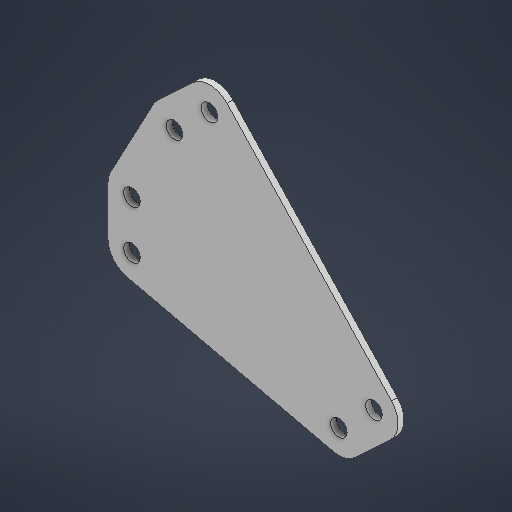
# Autodesk Inventor part: 2-Gearbox
Saved by Autodesk Inventor 2026.1 (Build 301233000, 233)
## iProperties
Created: 2025-08-06
Part Number: 2-Gearbox
Material: Generic
Document SubType Name: Modeling
Designer: roejo
Density: 1 g/cm^3
Appearance: Default
Author: roejo
Autodesk Inventor part; units mm, degrees
ref_plane "YZ Plane" through (0, 0, 0) normal (1, 0, 0) x (0, 1, 0)
ref_plane "XZ Plane" through (0, 0, 0) normal (0, 1, 0) x (-1, 0, 0)
ref_plane "XY Plane" through (0, 0, 0) normal (0, 0, 1) x (1, 0, 0)
sketch "Sketch1" plane through (0, 0, 0) normal (0, 0, 1) x (1, 0, 0)
  circle A0 centre (25.1062, -24.0271) radius 2.1844
  circle A1 centre (34.3733, -15.3432) radius 2.1844
  circle A2 centre (-18.3132, 22.3087) radius 2.1844
  circle A3 centre (-9.0461, 30.9926) radius 2.1844
  circle A4 centre (-29.4975, 1.3577) radius 2.1844
  circle A5 centre (-29.4975, -11.3423) radius 2.1844
  arc A6 (-35.0992, 4.3481) -> (-35.8475, 1.3577) centre (-29.4975, 1.3577) ccw
  arc A7 (-35.8475, -11.3423) -> (-30.9343, -17.5276) centre (-29.4975, -11.3423) ccw
  arc A8 (-22.6552, 26.9423) -> (-23.915, 25.2991) centre (-18.3132, 22.3087) ccw
  arc A9 (-4.4125, 35.3346) -> (-13.388, 35.6262) centre (-9.0461, 30.9926) ccw
  arc A10 (38.7153, -19.9767) -> (39.0069, -11.0012) centre (34.3733, -15.3432) ccw
  arc A11 (23.6693, -30.2123) -> (29.4481, -28.6606) centre (25.1062, -24.0271) ccw
  line L0 (38.7153, -19.9767) -> (29.4481, -28.6606)
  line L1 (-35.8475, -11.3423) -> (-35.8475, 1.3577)
  line L2 (-35.0992, 4.3481) -> (-23.915, 25.2991)
  line L3 (-4.4125, 35.3346) -> (39.0069, -11.0012)
  line L4 (-30.9343, -17.5276) -> (23.6693, -30.2123)
  line L5 (-22.6552, 26.9423) -> (-13.388, 35.6262)
  point P0 (0, 0)
  dimension "d0" = 12.7
  dimension "d1" = 12.7
  dimension "d2" = 12.7
  dimension "d3" = 12.7
  dimension "d4" = 12.7
  dimension "d5" = 12.7
  constraints: 12 centre point, 12 end point, 12 point on circle, 12 tangent, 6 coincident, 6 other
  measures "d0" diameter of A6
  measures "d1" diameter of A7
  measures "d2" diameter of A8
  measures "d3" diameter of A9
  measures "d4" diameter of A10
  measures "d5" diameter of A11
extrude "Extrusion1" add sketch "Sketch1" along normal blind 1.5875
body "Solid1"
